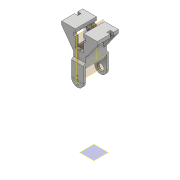
# Autodesk Inventor part: core_structure
Saved by Autodesk Inventor 2018 (Build 220112000, 112)
## iProperties
Created: 2018-02-12
Part Number: core_structure
Material: Generic
Document SubType Name: Modeling
Designer: Bardo91
Density: 1 g/cm^3
Appearance: Default
Author: Bardo91
Autodesk Inventor part; units mm, degrees
ref_plane "YZ Plane" through (0, 0, 0) normal (1, 0, 0) x (0, 1, 0)
ref_plane "XZ Plane" through (0, 0, 0) normal (0, 1, 0) x (-1, 0, 0)
ref_plane "XY Plane" through (0, 0, 0) normal (0, 0, 1) x (1, 0, 0)
sketch "Sketch1" plane through (0, 0, 0) normal (0, 0, 1) x (1, 0, 0)
  line L0 (0, 0) -> (18, 0)
  line L1 (18, 0) -> (18, 32)
  line L2 (18, 32) -> (0, 32)
  line L3 (0, 32) -> (0, 0)
  dimension "d0" = 18
  dimension "d1" = 32
  constraints: 8 end point, 2 perpendicular, 1 horizontal, 1 vertical
  measures "d0" distance of L0.start L0.end
  measures "d1" distance of L0.end L1.end
extrude "base" add sketch "Sketch1" along normal blind 25
sketch "Sketch2" plane through (0, 0, 25) normal (0, 0, 1) x (1, 0, 0)
  line L0 (18, 32) -> (0, 32) projected
  line L1 (9, 32) -> (9, 0)
  line L2 (9, 16) -> (9, 27.5)
  line L3 (9, 16) -> (20.5, 16) construction
  line L4 (9, 27.5) -> (15.25, 27.5)
  line L5 (15.25, 27.5) -> (15.25, 4.5)
  line L6 (15.25, 4.5) -> (2.75, 4.5)
  line L7 (2.75, 4.5) -> (2.75, 27.5)
  line L8 (2.75, 27.5) -> (9, 27.5)
  line L9 (0, 0) -> (18, 0) projected
  dimension "d4" = 11.5
  dimension "d5" = 90
  dimension "d6" = 6.25
  dimension "d7" = 23
  dimension "d8" = 12.5
  constraints: 16 end point, 6 perpendicular, 3 midpoint, 1 collinear, 1 horizontal, 1 point on line, 1 vertical
  measures "d4" distance of L2.start L2.end
  measures "d5" angle of L3 L2
  measures "d6" distance of L2.end L4.end
  measures "d7" distance of L4.end L5.end
  measures "d8" distance of L5.end L6.end
extrude "servo_place" cut sketch "Sketch2" against normal blind 18
sketch "Sketch3" plane through (0, 0, 25) normal (0, 0, 1) x (1, 0, 0)
  line L0 (2.75, 27.5) -> (15.25, 27.5) projected
  line L1 (9, 27.5) -> (9, 30.3)
  circle A0 centre (9, 30.3) radius 1
  line L2 (15.25, 4.5) -> (2.75, 4.5) projected
  line L3 (9, 4.5) -> (9, 1.7)
  circle A1 centre (9, 1.7) radius 1
  point P0 (0, 0)
  dimension "d11" = 2.8
  dimension "d12" = 2
  dimension "d13" = 2.8
  dimension "d14" = 2
  constraints: 4 end point, 2 centre point, 2 coincident, 2 midpoint, 2 vertical
  measures "d11" distance of L1.start L1.end
  measures "d12" diameter of A0
  measures "d13" distance of L3.start L3.end
  measures "d14" diameter of A1
extrude "screws_servo" cut sketch "Sketch3" against normal through all
ref_plane "Work Plane1" through (9, 22, -120) normal (0, 0, -1) x (-1, 0, 0)
sketch "Sketch6" plane through (0, 0, 25) normal (0, 0, 1) x (1, 0, 0)
  line L0 (0, 32) -> (0, 0) projected
  line L1 (2.75, 27.5) -> (15.25, 27.5) projected
  line L2 (0, 32) -> (2.75, 32)
  line L3 (2.75, 32) -> (2.75, 27.5)
  line L4 (2.75, 27.5) -> (0, 27.5)
  line L5 (0, 27.5) -> (0, 32)
  line L6 (18, 32) -> (15.2563, 32)
  line L7 (15.2563, 32) -> (15.2563, 27.5)
  line L8 (15.2563, 27.5) -> (18, 27.5)
  line L9 (18, 27.5) -> (18, 32)
  line L10 (15.25, 27.5) -> (15.25, 4.5) projected
  line L11 (18, 0) -> (15.25, 0)
  line L12 (15.25, 0) -> (15.25, 4.5)
  line L13 (15.25, 4.5) -> (18, 4.5)
  line L14 (18, 4.5) -> (18, 0)
  line L15 (0, 0) -> (2.75, 0)
  line L16 (2.75, 0) -> (2.75, 4.5)
  line L17 (2.75, 4.5) -> (0, 4.5)
  line L18 (0, 4.5) -> (0, 0)
  constraints: 32 end point, 8 parallel, 4 horizontal, 4 perpendicular, 4 point on line
extrude "pilars_top" add sketch "Sketch6" along normal blind 20
sketch "Sketch9" plane through (0, 0, 45) normal (0, 0, 1) x (1, 0, 0)
  line L0 (0, 32) -> (0, 0) projected
  line L1 (18, 0) -> (18, 32) projected
  line L2 (0, 32) -> (18, 32)
  line L3 (18, 32) -> (18, 0)
  line L4 (18, 0) -> (0, 0)
  line L5 (0, 0) -> (0, 32)
  line L6 (18, 32) -> (36, 32)
  line L7 (36, 32) -> (36, 0)
  line L8 (36, 0) -> (18, 0)
  line L9 (0, 32) -> (-18, 32)
  line L10 (-18, 32) -> (-18, 0)
  line L11 (-18, 0) -> (0, 0)
  point P0 (0, 22)
  point P1 (18, 22)
  dimension "d39" = 18
  dimension "d40" = 18
  constraints: 20 end point, 5 perpendicular, 3 parallel, 1 horizontal, 1 point on line, 1 vertical
  measures "d39" distance of L1.end L6.end
  measures "d40" distance of L0.start L9.end
extrude "base_top" add sketch "Sketch9" along normal blind 5
sketch "Sketch10" plane through (0, 0, 50) normal (0, 0, 1) x (1, 0, 0)
  line L0 (18, 32) -> (0, 32) projected
  line L1 (15.293, 32) -> (15.293, 0)
  line L2 (15.25, 27.5) -> (15.25, 4.5) projected
  line L3 (15.2563, 27.5) -> (15.2563, 32) projected
  line L4 (15.2563, 32) -> (2.7563, 32)
  line L5 (36, 32) -> (-18, 32) projected
  line L6 (2.7563, 32) -> (2.7563, 0)
  line L7 (0, 0) -> (18, 0) projected
  line L8 (15.293, 0) -> (2.7563, 0)
  dimension "d100" = 12.5
  constraints: 8 end point, 3 point on line, 1 collinear, 1 parallel, 1 perpendicular
  measures "d100" distance of L3.end L4.end
extrude "screw_hole" cut sketch "Sketch10" against normal blind 5
sketch "Sketch11" plane through (0, 0, 50) normal (0, 0, 1) x (1, 0, 0)
  circle A0 centre (9, 22) radius 6 projected
  line L0 (9, 22) -> (36, 22)
  line L1 (36, 0) -> (36, 32) projected
  line L2 (36, 22) -> (36, 24.5)
  line L3 (36, 24.5) -> (31, 24.5)
  line L4 (31, 24.5) -> (31, 19.5)
  line L5 (31, 19.5) -> (36, 19.5)
  line L6 (36, 19.5) -> (36, 24.5)
  line L7 (9, 22) -> (9, 34.0709)
  line L8 (-18, 22) -> (-18, 24.5)
  line L9 (-18, 24.5) -> (-13, 24.5)
  line L10 (-13, 24.5) -> (-13, 19.5)
  line L11 (-13, 19.5) -> (-18, 19.5)
  line L12 (-18, 19.5) -> (-18, 24.5)
  dimension "d60" = 2.5
  dimension "d61" = 5
  dimension "d62" = 5
  constraints: 24 end point, 5 symmetric about line, 3 perpendicular, 3 point on line, 1 collinear, 1 horizontal, 1 vertical
  measures "d60" distance of L0.end L2.end
  measures "d61" distance of L2.end L3.end
  measures "d62" distance of L3.end L4.end
extrude "Extrusion11" cut sketch "Sketch11" against normal blind 5 contours L4 L3 L1 L0 | L0 L1 L5 L4 | L8 L9 L10 L11 L12
ref_plane "Work Plane2" through (0, 0, 10) normal (0, 0, -1) x (-1, 0, 0)
sketch "Sketch12" plane through (0, 0, 10) normal (0, 0, -1) x (-1, 0, 0)
  line L0 (0, 0) -> (-18, 0) projected
  line L1 (-18, 0) -> (-18, -3)
  line L2 (-18, -3) -> (0, -3)
  line L3 (0, -3) -> (0, 0)
  line L4 (0, 0) -> (0, -3)
  line L5 (0, 0) -> (-18, 0)
  line L6 (-18, 32) -> (0, 32) projected
  line L7 (-18, 32) -> (0, 32)
  line L8 (0, 32) -> (0, 35)
  line L9 (0, 35) -> (-18, 35)
  line L10 (-18, 35) -> (-18, 32)
  dimension "d64" = 3
  dimension "d65" = 3
  constraints: 18 end point, 4 perpendicular, 3 collinear, 2 point on line, 1 vertical
  measures "d64" distance of L0.end L1.end
  measures "d65" distance of L6.end L8.end
extrude "connector_prev_servo" add sketch "Sketch12" along normal blind 32
chamfer "Chamfer2" distance 3 angle 45 2 edges at (9, 0, 10) (9, 32, 10)
fillet "Fillet3" radius 9 4 edges at (18, 33.5, -22) (0, 33.5, -22) (0, -1.5, -22) (18, -1.5, -22)
sketch "Sketch13" plane through (0, -3, 10) normal (0, -1, 0) x (1, 0, 0)
  arc A0 (0, -23) -> (18, -23) centre (9, -23) ccw projected
  circle A1 centre (9, -23) radius 1.75
  line L0 (9, -23) -> (15, -23)
  circle A2 centre (15, -23) radius 1
  circle A3 centre (9, -17) radius 1
  circle A4 centre (3, -23) radius 1
  circle A5 centre (9, -29) radius 1
  point P0 (0, -10)
  dimension "d72" = 3.5
  dimension "d73" = 6
  dimension "d74" = 2
  dimension "d77" = 360
  constraints: 5 centre point, 2 coincident, 2 end point, 1 horizontal, 9 other
  measures "d72" diameter of A1
  measures "d73" distance of L0.start L0.end
  measures "d74" diameter of A2
extrude "screw_holes" cut sketch "Sketch13" against normal up to surface (3 mm away)
fillet "Fillet4" radius 9 2 edges at (18, 16, 0) (0, 16, 0)
sketch "Sketch14" plane through (0, 35, 10) normal (0, 1, 0) x (1, 0, 0)
  arc A0 (18, 23) -> (0, 23) centre (9, 23) ccw projected
  circle A1 centre (9, 23) radius 5
  point P0 (0, 10)
  dimension "d82" = 10
  constraints: 1 centre point, 1 coincident
  measures "d82" diameter of A1
extrude "Extrusion14" cut sketch "Sketch14" against normal up to next
sketch "Sketch16" plane through (2.75, 0, 25) normal (0, -1, 0) x (1, 0, 0)
  line L0 (12.5063, 20) -> (15.25, 20) projected
  line L1 (15.25, 20) -> (33.25, 20)
  line L2 (15.25, 20) -> (15.25, -5)
  line L3 (15.25, -12) -> (15.25, 20) projected
  line L4 (15.25, -5) -> (33.25, 20)
  point P0 (-2.75, -25)
  dimension "d95" = 25
  constraints: 6 end point, 1 horizontal, 1 point on line
  measures "d95" distance of L0.end L2.end
extrude "Extrusion16" add sketch "Sketch16" against normal blind 4.6
ref_plane "Work Plane3" through (2.75, 16, 25) normal (0, 1, 0) x (1, 0, 0)
ref_plane "Work Plane4" through (9, -3, -13) normal (1, 0, 0) x (0, 0, -1)
mirror "Mirror1" about plane through (2.75, 16, 25) normal (0, 1, 0) of "Extrusion16"
mirror "Mirror2" about plane through (9, -3, -13) normal (1, 0, 0) of "Extrusion16", "Mirror1"
sketch "Sketch17" plane through (2.75, 32, 25) normal (0, 1, 0) x (1, 0, 0)
  line L0 (15.25, -20) -> (12.543, -20) projected
  line L1 (-2.75, -20) -> (15.25, -20)
  line L2 (15.25, -20) -> (15.25, -15)
  line L3 (15.25, 0) -> (15.25, -20) projected
  line L4 (15.25, -15) -> (-2.75, -15)
  line L5 (-2.75, -15) -> (-2.75, -20)
  point P0 (-2.75, 25)
  dimension "d101" = 5
  dimension "d104" = 18
  constraints: 8 end point, 2 perpendicular, 1 collinear, 1 point on line
  measures "d101" distance of L0.start L2.end
  measures "d104" distance of L1.start L0.start
extrude "Extrusion17" cut sketch "Sketch17" against normal through all
body "Solid1"
